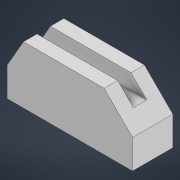
# Autodesk Inventor part: Pieza 5
Saved by Autodesk Inventor 2022 (Build 260153000, 153)
## iProperties
Created: 2022-06-27
Part Number: Pieza 5
Material: Genérico
Document SubType Name: Modeling
Designer: aleon
Density: 1 g/cm^3
Appearance: Valor por defecto
Author: aleon
Autodesk Inventor part; units mm, degrees
ref_plane "YZ Plane" through (0, 0, 0) normal (1, 0, 0) x (0, 1, 0)
ref_plane "XZ Plane" through (0, 0, 0) normal (0, 1, 0) x (-1, 0, 0)
ref_plane "XY Plane" through (0, 0, 0) normal (0, 0, 1) x (1, 0, 0)
sketch "Boceto1" plane through (0, 0, 0) normal (0, 0, 1) x (1, 0, 0)
  line L0 (-28, 0) -> (28, 0)
  line L1 (-28, 0) -> (-28, 13)
  line L2 (-28, 13) -> (-20.6795, 25.6795)
  line L3 (-20.6795, 25.6795) -> (15.3205, 25.6795)
  line L4 (15.3205, 25.6795) -> (28, 13)
  line L5 (28, 13) -> (28, 0)
  line L6 (15.3205, 25.6795) -> (15.3205, 18.6795)
  line L7 (-24.7209, 18.6795) -> (22.3205, 18.6795) construction
  point P0 (0, 0)
  dimension "d0" = 28
  dimension "d1" = 28
  dimension "d2" = 13
  dimension "d3" = 36
  dimension "d4" = 135
  dimension "d6" = 7
  dimension "d16" = 150
  constraints: 16 end point, 3 point on line, 2 horizontal, 2 vertical, 1 horizontal alignment, 1 parallel, 1 perpendicular
  measures "d0" distance of L0.end point (0, 0)
  measures "d1" distance of L0.start point (0, 0)
  measures "d2" vertical distance of L1.end L0.end
  measures "d3" distance of L2.end L3.end
  measures "d4" angle of L5 L4
  measures "d6" distance of L3.end L6.end
  measures "d16" angle of L2 L1
extrude "Extrusión1" add sketch "Boceto1" along normal mid plane 18
sketch "Boceto2" plane through (-20.6795, 25.6795, 9) normal (0, 1, 0) x (1, 0, 0)
  line L0 (-7.3205, 18) -> (-7.3205, 0) construction
  line L1 (-7.3205, 12) -> (48.6795, 12) construction
  line L2 (48.6795, 18) -> (48.6795, 0) construction
  line L3 (-7.3205, 6) -> (48.6795, 6) construction
  line L4 (0, 18) -> (36, 18) construction
  line L5 (-4.0415, 12) -> (-4.0415, 6)
  line L6 (43, 12) -> (43, 6)
  line L7 (-4.0415, 12) -> (43, 12)
  line L8 (43, 6) -> (-4.0415, 6)
  point P0 (20.6795, 9)
  point P1 (-4.0415, 9)
  point P2 (43, 9)
  dimension "d9" = 6
  dimension "d10" = 6
  constraints: 12 end point, 6 point on line, 2 collinear, 2 horizontal, 2 perpendicular
  measures "d9" distance between parallel lines of L1 L4
  measures "d10" distance between parallel lines of L3 L1
extrude "Extrusión2" cut sketch "Boceto2" against normal blind 7
